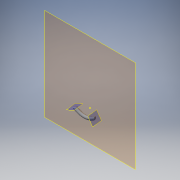
# Autodesk Inventor part: Wire3
Saved by Autodesk Inventor 2018 (Build 220112000, 112)
## iProperties
Created: 2018-06-11
Part Number: Wire3
Material: Generic
Document SubType Name: Modeling
Designer: DPLXuser
Density: 1 g/cm^3
Appearance: Default
Author: DPLXuser
Autodesk Inventor part; units mm, degrees
ref_plane "YZ Plane" through (0, 0, 0) normal (1, 0, 0) x (0, 1, 0)
ref_plane "XZ Plane" through (0, 0, 0) normal (0, 1, 0) x (-1, 0, 0)
ref_plane "XY Plane" through (0, 0, 0) normal (0, 0, 1) x (1, 0, 0)
ref_plane "Work Plane1" through (0, 0, 0) normal (0.4228, -0.9, -0.1061) x (0.9048, 0.4258, -0.0066)
sketch "Sketch1" plane through (0, 0, 0) normal (0.4228, -0.9, -0.1061) x (0.9048, 0.4258, -0.0066)
  circle A0 centre (0, 0) radius 6.35
  dimension "d0" = 12.7
  constraints: 1 centre point, 1 coincident
  measures "d0" diameter of A0
ref_plane "Work Plane2" through (77.6105, 0, 0) normal (-0.9062, -0.4199, -0.0495) x (-0.4228, 0.9, 0.1061)
sketch "Sketch2" plane through (77.6105, 0, 0) normal (-0.9062, -0.4199, -0.0495) x (-0.4228, 0.9, 0.1061)
  point P0 (32.8115, 0)
ref_plane "Work Plane3" through (0, 0, 0) normal (0, 0, 1) x (1, 0, 0)
sketch "Sketch3" plane through (0, 0, 0) normal (0, 0, 1) x (1, 0, 0)
  spline S0 degree 2 poles (0, 0) (40.2857, -24.9889) (77.6688, 0) knots 0 0 0 1 1 1
  point P0 (40.1611, -12.4914)
  constraints: 3 other
sweep "Sweep1" add profiles "Sketch1" path "Sketch3"
body "Solid1"
